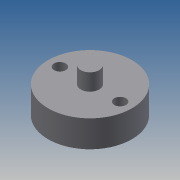
# Autodesk Inventor part: stopper
Saved by Autodesk Inventor 2013 (Build 170138000, 138)
## iProperties
Created: 2017-03-30
Part Number: stopper
Material: Generic
Document SubType Name: Modeling
Designer: employee
Density: 1 g/cm^3
Author: employee
Autodesk Inventor part; units mm, degrees
ref_plane "YZ Plane" through (0, 0, 0) normal (1, 0, 0) x (0, 1, 0)
ref_plane "XZ Plane" through (0, 0, 0) normal (0, 1, 0) x (-1, 0, 0)
ref_plane "XY Plane" through (0, 0, 0) normal (0, 0, 1) x (1, 0, 0)
sketch "Sketch1" plane through (0, 0, 0) normal (0, 0, 1) x (1, 0, 0)
  circle A0 centre (0, 0) radius 12.5
  dimension "d0" = 25
  constraints: 1 centre point, 1 coincident
  measures "d0" diameter of A0
extrude "Extrusion1" add sketch "Sketch1" along normal blind 8
sketch "Sketch2" plane through (0, 0, 8) normal (0, 0, 1) x (1, 0, 0)
  circle A0 centre (0, 0) radius 12.5 projected
  circle A1 centre (0, 0) radius 2.75
  dimension "d4" = 5.5
  constraints: 1 centre point, 1 coincident
  measures "d4" diameter of A1
extrude "Extrusion2" add sketch "Sketch2" along normal blind 5 contours A1
sketch "Sketch3" plane through (0, 0, 8) normal (0, 0, 1) x (1, 0, 0)
  circle A0 centre (0, 0) radius 2.75 projected
  circle A1 centre (-7.5, 0) radius 1.75
  circle A2 centre (7.5, 0) radius 1.75
  dimension "d8" = 7.5
  dimension "d9" = 7.5
  dimension "d10" = 3.5
  constraints: 2 centre point, 2 horizontal alignment, 1 equal radius
  measures "d8" distance of A2.centre A0.centre
  measures "d9" distance of A0.centre A1.centre
  measures "d10" diameter of A1
extrude "Extrusion3" cut sketch "Sketch3" against normal through all contours A1 | A2
sketch "Sketch4" plane through (0, 0, 0) normal (0, 0, -1) x (-1, 0, 0)
  circle A0 centre (7.5, 0) radius 1.75 projected
  circle A1 centre (-7.5, 0) radius 1.75 projected
  line L0 (-7.5, 3.1754) -> (-4.75, 1.5877)
  line L1 (-4.75, 1.5877) -> (-4.75, -1.5877)
  line L2 (-4.75, -1.5877) -> (-7.5, -3.1754)
  line L3 (-7.5, -3.1754) -> (-10.25, -1.5877)
  line L4 (-10.25, -1.5877) -> (-10.25, 1.5877)
  line L5 (-10.25, 1.5877) -> (-7.5, 3.1754)
  line L6 (7.5, 3.1754) -> (10.25, 1.5877)
  line L7 (10.25, 1.5877) -> (10.25, -1.5877)
  line L8 (10.25, -1.5877) -> (7.5, -3.1754)
  line L9 (7.5, -3.1754) -> (4.75, -1.5877)
  line L10 (4.75, -1.5877) -> (4.75, 1.5877)
  line L11 (4.75, 1.5877) -> (7.5, 3.1754)
  dimension "d13" = 5.5
  constraints: 24 end point, 2 coincident, 2 vertical, 1 parallel, 26 other
  measures "d13" distance between parallel lines of L7 L10
extrude "Extrusion4" cut sketch "Sketch4" against normal blind 4
chamfer "Chamfer2" distance 2 angle 45 1 edges at (-12.5, 0, 0)
body "Solid1"
